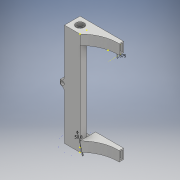
# Autodesk Inventor part: frontAxelHolder 11-28
Saved by Autodesk Inventor 2018 (Build 220112000, 112)
## iProperties
Created: 2019-11-28
Part Number: frontAxelHolder 11-28
Material: Generic
Document SubType Name: Modeling
Designer: Aditya Kendre
Density: 1 g/cm^3
Appearance: Default
Author: Aditya Kendre
Autodesk Inventor part; units mm, degrees
ref_plane "YZ Plane" through (0, 0, 0) normal (1, 0, 0) x (0, 1, 0)
ref_plane "XZ Plane" through (0, 0, 0) normal (0, 1, 0) x (-1, 0, 0)
ref_plane "XY Plane" through (0, 0, 0) normal (0, 0, 1) x (1, 0, 0)
sketch "Sketch1" plane through (0, 0, 0) normal (0, 1, 0) x (-1, 0, 0)
  line L0 (0, 0) -> (25, 0)
  line L1 (25, 0) -> (25, -165)
  line L2 (25, -165) -> (0, -165)
  line L3 (0, -165) -> (0, 0)
  dimension "d0" = 25
  dimension "d1" = 165
  constraints: 8 end point, 2 parallel, 1 horizontal, 1 perpendicular
  measures "d0" distance of L1.end L2.end
  measures "d1" distance of L0.end L1.end
extrude "Extrusion1" add sketch "Sketch1" along normal blind 3
sketch "Sketch2" plane through (0, 3, 0) normal (0, 1, 0) x (1, 0, 0)
  line L0 (-25, 165) -> (-25, 0) projected
  line L1 (0, 0) -> (0, 165) projected
  line L2 (-25, 0) -> (0, 0)
  line L3 (0, 0) -> (0, 7)
  line L4 (0, 7) -> (-25, 7)
  line L5 (-25, 7) -> (-25, 0)
  line L6 (0, 165) -> (-25, 165) projected
  line L7 (-25, 165) -> (0, 165)
  line L8 (0, 165) -> (0, 158)
  line L9 (0, 158) -> (-25, 158)
  line L10 (-25, 158) -> (-25, 165)
  dimension "d4" = 7
  dimension "d5" = 7
  constraints: 16 end point, 4 parallel, 2 horizontal, 2 perpendicular, 2 point on line
  measures "d4" distance of L3.end L2.end
  measures "d5" distance of L7.end L8.end
extrude "Extrusion2" add sketch "Sketch2" along normal blind 22 contours L6 L1 L9 L0 | L4 L1 L2 L0
sketch "Sketch3" plane through (-25, 0, 0) normal (0, 0, 1) x (1, 0, 0)
  point P0 (25, 0)
sketch "Sketch4" plane through (-25, 0, 0) normal (0, 0, 1) x (1, 0, 0)
  line L0 (25, 25) -> (0, 25) construction
  line L1 (25, 0) -> (0, 25) construction
  circle A0 centre (12.5, 12.5) radius 6.5
  dimension "d8" = 13
  constraints: 2 end point, 1 centre point, 1 coincident, 1 midpoint
  measures "d8" diameter of A0
extrude "Extrusion3" cut sketch "Sketch4" against normal blind 5
sketch "Sketch5" plane through (0, 0, -165) normal (0, 0, -1) x (-1, 0, 0)
  circle A0 centre (12.5, 12.5) radius 6.5 projected
  circle A1 centre (12.5, 12.5) radius 6.5
  point P0 (0, 0)
  constraints: 1 centre point, 1 coincident
extrude "Extrusion4" cut sketch "Sketch5" against normal blind 5
sketch "Sketch6" plane through (-25, 0, 0) normal (0, 0, 1) x (1, 0, 0)
  circle A0 centre (12.5, 12.5) radius 6.5 projected
  circle A1 centre (12.5, 12.5) radius 5
  point P0 (25, 0)
  dimension "d13" = 10
  constraints: 1 centre point, 1 coincident
  measures "d13" diameter of A1
extrude "Extrusion5" cut sketch "Sketch6" against normal blind 165 contours A1
sketch "Sketch7" plane through (-25, 3, -158) normal (0, 0, 1) x (1, 0, 0)
  line L0 (25, 0) -> (25, 22) construction
  line L1 (0, 0) -> (0, 22) construction
  point P0 (25, -3)
sketch "Sketch8" plane through (-25, 3, -158) normal (0, 0, 1) x (1, 0, 0)
  circle A0 centre (12.5, 9.5) radius 5 projected
  point P0 (25, -3)
  constraints: 1 coincident
sketch "Sketch9" plane through (0, 3, 0) normal (0, 1, 0) x (1, 0, 0)
  line L0 (-25, 158) -> (0, 158) projected
  line L1 (0, 7) -> (-25, 7) projected
  line L2 (-25, 158) -> (-20, 158)
  line L3 (-20, 158) -> (-20, 7)
  line L4 (-20, 7) -> (-25, 7)
  line L5 (-25, 7) -> (-25, 158)
  line L6 (0, 0) -> (0, 7) projected
  line L7 (0, 7) -> (-5, 7)
  line L8 (-5, 7) -> (-5, 158)
  line L9 (-5, 158) -> (0, 158)
  line L10 (0, 158) -> (0, 7)
  dimension "d16" = 5
  dimension "d17" = 5
  constraints: 16 end point, 4 parallel, 2 horizontal, 2 perpendicular, 2 point on line
  measures "d16" distance of L3.end L4.end
  measures "d17" distance of L8.end L9.end
extrude "Extrusion6" add sketch "Sketch9" along normal blind 7.5 contours L0 L3 L1 L5 | L0 L10 L1 L8
fillet "Fillet1" radius 2 2 edges at (-5, 10.5, -82.5) (-20, 10.5, -82.5)
sketch "Sketch10" plane through (0, 0, 0) normal (1, 0, 0) x (0, 0, -1)
  line L0 (0, 0) -> (0, 25) projected
  line L1 (165, 0) -> (0, 0) projected
  line L2 (0, 25) -> (16, 25)
  line L3 (16, 25) -> (16, 0)
  line L4 (16, 0) -> (0, 0)
  line L5 (0, 0) -> (0, 25)
  line L6 (165, 0) -> (165, 25) projected
  line L7 (165, 25) -> (149, 25)
  line L8 (149, 25) -> (149, 0)
  line L9 (149, 0) -> (165, 0)
  line L10 (165, 0) -> (165, 25)
  dimension "d21" = 16
  dimension "d22" = 16
  constraints: 16 end point, 4 parallel, 2 horizontal, 2 perpendicular, 2 point on line
  measures "d21" distance of L3.end L4.end
  measures "d22" distance of L9.end L8.end
extrude "Extrusion7" add sketch "Sketch10" along normal blind 45
sketch "Sketch11" plane through (45, 0, 0) normal (1, 0, 0) x (0, 0, -1)
  line L0 (7, 25) -> (0, 25) construction
  line L1 (16, 0) -> (16, 25) construction
  line L2 (0, 25) -> (16, 25) construction
  line L3 (16, 25) -> (7, 25) construction
  line L4 (8, 25) -> (8, 21.5) construction
  line L5 (14.125, 19.875) -> (1.875, 19.875)
  line L6 (1.875, 19.875) -> (1.875, 23.125)
  line L7 (1.875, 23.125) -> (14.125, 23.125)
  line L8 (14.125, 23.125) -> (14.125, 19.875)
  line L9 (14.125, 19.875) -> (1.875, 23.125) construction
  line L10 (1.875, 19.875) -> (14.125, 23.125) construction
  line L11 (165, 25) -> (149, 25) construction
  line L12 (157, 25) -> (157, 21.5) construction
  line L13 (163.125, 19.875) -> (150.875, 19.875)
  line L14 (150.875, 19.875) -> (150.875, 23.125)
  line L15 (150.875, 23.125) -> (163.125, 23.125)
  line L16 (163.125, 23.125) -> (163.125, 19.875)
  line L17 (163.125, 19.875) -> (150.875, 23.125) construction
  line L18 (150.875, 19.875) -> (163.125, 23.125) construction
  point P0 (0, 0)
  dimension "d25" = 3.5
  dimension "d26" = 12.25
  dimension "d27" = 3.25
  dimension "d28" = 3.5
  dimension "d29" = 12.25
  dimension "d30" = 3.25
  constraints: 30 end point, 5 midpoint, 4 parallel, 3 horizontal, 3 perpendicular, 1 point on line, 1 vertical
  measures "d25" distance of L4.start L4.end
  measures "d26" distance of L6.end L7.end
  measures "d27" distance of L5.end L6.end
  measures "d28" distance of L12.start L12.end
  measures "d29" distance of L14.end L15.end
  measures "d30" distance of L13.end L14.end
extrude "Extrusion8" cut sketch "Sketch11" against normal blind 40
sketch "Sketch12" plane through (45, 0, 0) normal (1, 0, 0) x (0, 0, -1)
  line L0 (16, 0) -> (16, 25) construction
  line L1 (0, 19.875) -> (16, 19.875) construction
  line L2 (16, 19.875) -> (16, 18) construction
  line L3 (16, 18) -> (0, 18) construction
  line L4 (0, 18) -> (0, 19.875) construction
  point P0 (0, 0)
  dimension "d33" = 1.875
  constraints: 8 end point, 2 parallel, 1 horizontal, 1 perpendicular, 1 point on line
  measures "d33" distance of L1.end L2.end
sketch "Sketch13" plane through (-25, 0, 0) normal (0, 0, 1) x (1, 0, 0)
  line L0 (70, 0) -> (70, 25) construction
  line L1 (70, 25) -> (70, 18) construction
  arc A0 (70, 18) -> (25, 0) centre (67.8851, -41.9627) ccw
  line L2 (70, 25) -> (70, 0) projected
  line L3 (70, 18) -> (70, 0)
  line L4 (70, 0) -> (25, 0)
  dimension "d34" = 7
  dimension "d35" = 60
  constraints: 6 end point, 2 point on circle, 1 centre point, 1 collinear, 1 perpendicular, 1 point on line
  measures "d34" distance of L0.end L1.end
  measures "d35" radius of A0
extrude "Extrusion9" cut sketch "Sketch13" against normal blind 165
sketch "Sketch14" plane through (0, 10.5, 0) normal (0, 1, 0) x (1, 0, 0)
  point P0 (0, 0)
sketch "Sketch15" plane through (-25, 0, -165) normal (0, 0, -1) x (-1, 0, 0)
  circle A0 centre (-12.5, 12.5) radius 6.5 construction
  circle A1 centre (-12.5, 12.5) radius 25.4 construction
  point P0 (-25, 0)
  dimension "d38" = 50.8
  constraints: 1 centre point, 1 coincident
  measures "d38" diameter of A1
sketch "Sketch16" plane through (0, 10.5, 0) normal (0, 1, 0) x (1, 0, 0)
  line L0 (-25, 0) -> (-25, 165) projected
  line L1 (-25, 82.5) -> (-32, 82.5)
  line L2 (-32, 82.5) -> (-32, 86)
  line L3 (-32, 86) -> (-25, 86)
  line L4 (-25, 86) -> (-25, 82.5)
  line L5 (-32, 82.5) -> (-25, 82.5)
  line L6 (-25, 82.5) -> (-25, 79)
  line L7 (-25, 79) -> (-32, 79)
  line L8 (-32, 79) -> (-32, 82.5)
  point P0 (0, 0)
  dimension "d39" = 7
  dimension "d40" = 3.5
  dimension "d41" = 3.5
  constraints: 16 end point, 4 parallel, 2 horizontal, 2 perpendicular, 1 midpoint, 1 point on line
  measures "d39" distance of L2.end L3.end
  measures "d40" distance of L1.end L2.end
  measures "d41" distance of L5.end L6.end
extrude "Extrusion10" add sketch "Sketch16" against normal blind 10.5
sketch "Sketch17" plane through (0, 10.5, 0) normal (0, 1, 0) x (1, 0, 0)
  line L0 (-32, 79) -> (-25, 79) construction
  line L1 (-25, 86) -> (-32, 86) construction
  line L2 (-25, 79) -> (-32, 86) construction
  circle A0 centre (-28.5, 82.5) radius 3.175
  point P0 (0, 0)
  dimension "d44" = 6.35
  constraints: 2 end point, 1 centre point, 1 midpoint
  measures "d44" diameter of A0
extrude "Extrusion11" cut sketch "Sketch17" against normal blind 10.5
fillet "Fillet2" radius 7 2 edges at (-25, 5.25, -79) (-25, 5.25, -86)
body "Solid1"
